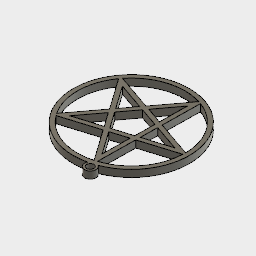
pendent (Autodesk Fusion 360 design; units mm, degrees)
Autodesk Fusion 360 part; units mm, degrees
sketch "草图1" plane through (0, 0, 0) normal (0, 1, 0) x (1, 0, 0)
  line L0 (-31.312, -20.8341) -> (-15.5098, 0.2355)
  line L1 (-30.1855, -22.4353) -> (-5.0168, -14.6779)
  line L2 (-5.0168, -14.6779) -> (10.1385, -36.2176)
  line L3 (12.4093, -9.307) -> (12.0094, -35.641)
  line L4 (12.6861, 8.9259) -> (37.6077, 0.408)
  circle A0 centre (0, 0) radius 40.6099
  arc A1 (-30.6651, 21.7752) -> (-31.312, -20.8341) centre (0, 0) ccw
  arc A2 (-30.1855, -22.4353) -> (10.1385, -36.2176) centre (0, 0) ccw
  arc A3 (12.0094, -35.641) -> (37.578, -1.5496) centre (0, 0) ccw
  arc A4 (37.6077, 0.408) -> (13.086, 35.2599) centre (0, 0) ccw
  arc A5 (11.2334, 35.8931) -> (-29.4904, 23.3414) centre (0, 0) ccw
  line L5 (-13.6172, 2.759) -> (-6.4615, 12.3)
  line L6 (-4.5688, 14.8235) -> (11.2334, 35.8931)
  line L7 (-29.4904, 23.3414) -> (-4.5688, 14.8235)
  line L8 (-1.584, 13.8033) -> (9.7013, 9.9461)
  line L9 (-24.7214, 18.541) -> (-6.4615, 12.3)
  line L10 (-1.584, 13.8033) -> (9.9942, 29.2409)
  line L11 (13.086, 35.2599) -> (12.6861, 8.9259)
  line L12 (12.6382, 5.7719) -> (12.4572, -6.1529)
  line L13 (9.9942, 29.2409) -> (9.7013, 9.9461)
  line L14 (12.4572, -6.1529) -> (30.8981, -0.4691)
  line L15 (-2.0023, -13.7488) -> (9.3948, -10.2361)
  line L16 (12.4093, -9.307) -> (37.578, -1.5496)
  line L17 (9.6534, 6.7921) -> (9.4427, -7.082)
  line L18 (9.3948, -10.2361) -> (9.1019, -29.5309)
  line L19 (-3.4766, 11.2798) -> (9.6534, 6.7921)
  line L20 (12.6382, 5.7719) -> (30.8981, -0.4691)
  line L21 (-24.7214, 18.541) -> (-13.6172, 2.759)
  line L22 (-11.802, 0.1792) -> (-3.8175, -11.169)
  line L23 (-2.0023, -13.7488) -> (9.1019, -29.5309)
  line L24 (-30.6651, 21.7752) -> (-15.5098, 0.2355)
  line L25 (-13.6947, -2.3443) -> (-6.8319, -12.0981)
  line L26 (-25.2729, -17.7819) -> (-13.6947, -2.3443)
  line L27 (-11.802, 0.1792) -> (-3.4766, 11.2798)
  line L28 (-25.2729, -17.7819) -> (-6.8319, -12.0981)
  line L29 (-3.8175, -11.169) -> (9.4427, -7.082)
extrude "拉伸1" add sketch "草图1" along normal blind 5 makes body 1
cylinder "圆柱体基本要素1" add diameter 8 height 5 placed x (1, 0, 0) y (0, 0, -1) z (0, 1, 0) at (14, 0, 66) separate body makes body 2
cylinder "圆柱体基本要素2" add diameter 5 height 5 placed x (1, 0, 0) y (0, 0, -1) z (0, 1, 0) at (14, 5, 66) bodies 2
move_face "偏移面1" offset -10 1 faces at (13.4804, 10, 65.5179) on bodies 2
cylinder "圆柱体基本要素3" add diameter 5 height 5 placed x (1, 0, 0) y (0, 0, -1) z (0, 1, 0) at (5, 0, 58) separate body makes body 3
move_body "对齐1" bodies 2 to x (1, 0, 0) y (0, 1, 0) z (0, 0, 1) at (-9, 0, -8)
combine "合并1" operation cut target body 2 tool bodies 3
move_body "移动1" bodies 2 to x (1, 0, 0) y (0, 1, 0) z (0, 0, 1) at (7.5748, 0, -16.7519)
combine "合并2" operation add target body 1 tool bodies 2
